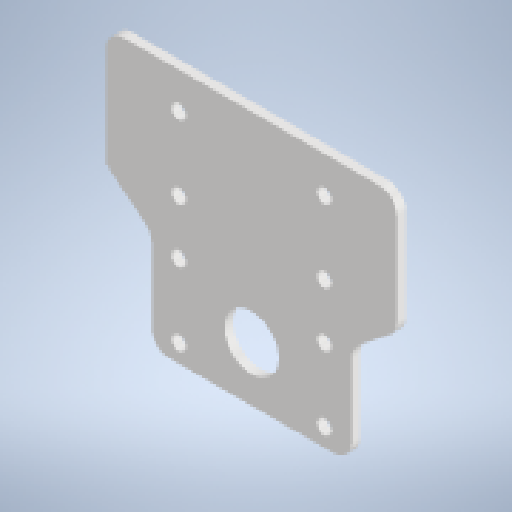
# Autodesk Inventor part: Dipper Plate
Saved by Autodesk Inventor 2023 (Build 270158000, 158)
## iProperties
Created: 2023-03-02
Part Number: Dipper Plate
Material: Generic
Document SubType Name: Modeling
Designer: Gabriel - T3 CAD
Density: 1 g/cm^3
Appearance: Default
Author: Gabriel - T3 CAD
Autodesk Inventor part; units mm, degrees
ref_plane "YZ Plane" through (0, 0, 0) normal (1, 0, 0) x (0, 1, 0)
ref_plane "XZ Plane" through (0, 0, 0) normal (0, 1, 0) x (-1, 0, 0)
ref_plane "XY Plane" through (0, 0, 0) normal (0, 0, 1) x (1, 0, 0)
sketch "Sketch1" plane through (0, 0, 0) normal (0, 0, 1) x (1, 0, 0)
  line L0 (0, 0) -> (-101.6, 0)
  line L1 (-101.6, 0) -> (-101.6, 101.6)
  line L2 (-95.25, 101.6) -> (0, 101.6)
  circle A0 centre (-76.2, 88.9) radius 2.5797
  circle A1 centre (-76.2, 63.5) radius 2.5797
  circle A2 centre (-25.4, 88.9) radius 2.5797
  circle A3 centre (-25.4, 63.5) radius 2.5797
  circle A4 centre (-50.8, 19.05) radius 9.525
  circle A5 centre (-76.2, 31.75) radius 2.5797
  circle A6 centre (-76.2, 6.35) radius 2.5797
  circle A7 centre (-25.4, 31.75) radius 2.5797
  circle A8 centre (-25.4, 6.35) radius 2.5797
  line L3 (-22.225, 0) -> (-79.375, 0)
  line L4 (-101.6, 50.677) -> (-101.6, 95.25)
  line L5 (-101.6, 101.6) -> (-6.35, 101.6)
  line L6 (0, 0) -> (-15.875, 0)
  line L7 (-15.875, 6.35) -> (-15.875, 31.873)
  line L8 (-101.6, 0) -> (-85.725, 0)
  line L9 (-85.725, 6.35) -> (-85.725, 31.873)
  line L10 (-85.725, 47.625) -> (-101.6, 47.625)
  line L11 (-101.6, 47.625) -> (-101.6, 0)
  line L12 (-101.6, 47.625) -> (-88.8573, 47.625)
  line L13 (-101.6, 26.0622) -> (-101.6, 47.625)
  line L14 (0, 95.25) -> (0, 50.677)
  line L15 (-15.875, 47.625) -> (0, 47.625)
  line L16 (-15.875, 47.625) -> (0, 47.625)
  line L17 (0, 47.625) -> (0, 34.925)
  line L18 (0, 34.925) -> (-15.875, 34.925)
  line L19 (-15.875, 34.925) -> (-15.875, 47.625)
  line L20 (-85.725, 47.625) -> (-101.6, 47.625)
  line L21 (-101.6, 47.625) -> (-101.6, 34.925)
  line L22 (-101.6, 34.925) -> (-85.725, 34.925)
  line L23 (-85.725, 34.925) -> (-85.725, 47.625)
  line L24 (-101.6, 41.275) -> (-85.725, 41.275)
  line L25 (-13.4918, 36.8315) -> (-2.3832, 45.7185)
  line L26 (-88.1082, 36.8315) -> (-99.2168, 45.7185)
  arc A9 (-101.6, 50.677) -> (-99.2168, 45.7185) centre (-95.25, 50.677) ccw
  arc A10 (-85.725, 31.873) -> (-88.1082, 36.8315) centre (-92.075, 31.873) ccw
  arc A11 (-2.3832, 45.7185) -> (0, 50.677) centre (-6.35, 50.677) ccw
  arc A12 (-13.4918, 36.8315) -> (-15.875, 31.873) centre (-9.525, 31.873) ccw
  arc A13 (-22.225, 0) -> (-15.875, 6.35) centre (-22.225, 6.35) ccw
  arc A14 (-85.725, 6.35) -> (-79.375, 0) centre (-79.375, 6.35) ccw
  arc A15 (0, 95.25) -> (-6.35, 101.6) centre (-6.35, 95.25) ccw
  arc A16 (-95.25, 101.6) -> (-101.6, 95.25) centre (-95.25, 95.25) ccw
  point P0 (0, 101.6)
  point P1 (0, 88.9)
  point P2 (-100.8185, 47.625)
  point P3 (-6.35, 101.6)
  point P4 (-101.6, 95.25)
  point P5 (-95.25, 101.6)
  dimension "d0" = 101.6
  dimension "d1" = 101.6
  dimension "d4" = 25.4
  dimension "d7" = 50.8
  dimension "d10" = 12.7
  dimension "d11" = 25.4
  dimension "d12" = 5.1594
  dimension "d13" = 19.05
  dimension "d14" = 5.1594
  dimension "d17" = 25.4
  dimension "d20" = 50.8
  dimension "d23" = 25.4
  dimension "d24" = 6.35
  dimension "d26" = 50.8
  dimension "d29" = 12.7
  dimension "d30" = 101.6
  dimension "d31" = 101.6
  dimension "d32" = 15.875
  dimension "d34" = 101.6
  dimension "d35" = 12.7
  dimension "d36" = 41.275
  dimension "d37" = 6.35
  dimension "d38" = 6.35
  dimension "d39" = 6.35
  dimension "d40" = 88.8572
  dimension "d41" = 21.5628
  dimension "d42" = 6.35
  constraints: 54 end point, 18 point on line, 17 centre point, 16 point on circle, 16 tangent, 9 horizontal, 9 perpendicular, 8 parallel, 4 equal length, 4 equal radius, 2 midpoint, 2 vertical, 12 other
  measures "d0" distance of L1.end L2.end
  measures "d1" distance of L0.end L1.end
  measures "d4" distance of A0.centre A1.centre
  measures "d7" distance of A0.centre A2.centre
  measures "d10" distance from line of L2 A0.centre
  measures "d11" distance from line of L1 A0.centre
  measures "d12" diameter of A0
  measures "d13" diameter of A4
  measures "d14" diameter of A5
  measures "d17" distance of A5.centre A6.centre
  measures "d20" distance of A5.centre A7.centre
  measures "d23" distance from line of L1 A5.centre
  measures "d24" distance from line of L0 A6.centre
  measures "d26" distance from line of L1 A4.centre
  measures "d29" vertical distance of A6.centre A4.centre
  measures "d30" distance of L1.end point (0, 101.6)
  measures "d31" distance of L8.start L1.end
  measures "d32" distance of L10.start L10.end
  measures "d34" distance of L0.start L0.end
  measures "d35" distance of L20.end L21.end
  measures "d36" distance between parallel lines of L0 L24
  measures "d37" radius of A9
  measures "d38" radius of A13
  measures "d39" radius of A14
  measures "d40" distance from line of L12.end L17
  measures "d41" distance from line of L13.start L15
  measures "d42" radius of A15
extrude "Extrusion1" add sketch "Sketch1" along normal blind 3.175 contours L0 A14 L9 A10 L22 L23 L10 A9 L1 A16 L2 A15 L14 A11 L15 L19 L18 A12 L7 A13 | L18 L19 L15 A11 L25 A12 | A10 L26 L24 L23 L22 | L24 L26 A9 L10 L23 | L1 A9 L10
body "Solid1"
